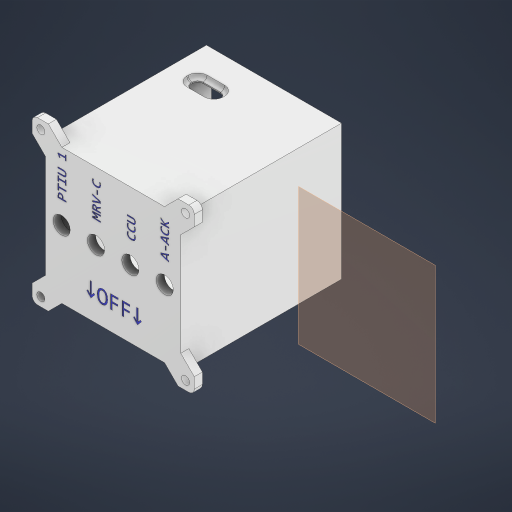
# Autodesk Inventor part: casing_1x1_lvl3
Saved by Autodesk Inventor 2024 (Build 280153000, 153)
## iProperties
Created: 2026-04-07
Part Number: casing_1x1_lvl3
Material: ABS Plastic
Document SubType Name: Modeling
Designer: schar
Density: 1.06 g/cm^3
Appearance: Smooth - White
Author: schar
Autodesk Inventor part; units mm, degrees
ref_plane "YZ Plane" through (0, 0, 0) normal (1, 0, 0) x (0, 1, 0)
sketch "Sketch1" plane through (0, 0, 0) normal (0, 0, 1) x (1, 0, 0)
  line L0 (51.6317, -54.9773) -> (91.6317, -54.9773) projected
  line L1 (85.3617, -57.4773) -> (85.3617, -57.6773) projected
  line L2 (48.6317, -97.9773) -> (48.6317, -57.9773) projected
  line L3 (91.6317, -100.9773) -> (51.6317, -100.9773) projected
  line L4 (48.6317, -77.9773) -> (85.3617, -57.5773)
  line L5 (71.6317, -54.9773) -> (71.6317, -100.9773)
  line L6 (48.5522, -54.8773) -> (94.7112, -54.8773)
  line L7 (94.7112, -54.8773) -> (94.7112, -101.0773)
  line L8 (94.7112, -101.0773) -> (48.5522, -101.0773)
  line L9 (48.5522, -101.0773) -> (48.5522, -54.8773)
  line L10 (48.5522, -54.8773) -> (94.7112, -101.0773) construction
  line L11 (94.7112, -54.8773) -> (48.5522, -101.0773) construction
  line L12 (46.6317, -52.9773) -> (96.6317, -52.9773)
  line L13 (96.6317, -52.9773) -> (96.6317, -102.9773)
  line L14 (96.6317, -102.9773) -> (46.6317, -102.9773)
  line L15 (46.6317, -102.9773) -> (46.6317, -52.9773)
  line L16 (46.6317, -52.9773) -> (96.6317, -102.9773) construction
  line L17 (96.6317, -52.9773) -> (46.6317, -102.9773) construction
  line L18 (36.6317, -42.9773) -> (106.6317, -42.9773)
  line L19 (106.6317, -42.9773) -> (106.6317, -112.9773)
  line L20 (106.6317, -112.9773) -> (36.6317, -112.9773)
  line L21 (36.6317, -112.9773) -> (36.6317, -42.9773)
  line L22 (36.6317, -42.9773) -> (106.6317, -112.9773) construction
  line L23 (106.6317, -42.9773) -> (36.6317, -112.9773) construction
  point P0 (0, 0)
  point P1 (71.6317, -77.9773)
  dimension "d0" = 46.159
  dimension "d1" = 46.2
  dimension "d2" = 50
  dimension "d3" = 50
  dimension "d4" = 70
  dimension "d5" = 70
  constraints: 40 end point, 11 midpoint, 6 parallel, 3 horizontal, 3 perpendicular
  measures "d0" distance of L7.end L8.end
  measures "d1" distance of L6.end L7.end
  measures "d2" distance of L13.end L14.end
  measures "d3" distance of L12.end L13.end
  measures "d4" distance of L19.end L20.end
  measures "d5" distance of L18.end L19.end
extrude "Extrusion1" add sketch "Sketch1" along normal blind 40 and the other way blind 30 contours L12 L13 L14 L15
ref_plane "Work Plane1" through (0, 0, 0) normal (0, 0, 1) x (1, 0, 0)
sketch "Sketch2" plane through (0, 0, 0) normal (0, 0, 1) x (1, 0, 0)
  line L0 (85.3617, -57.4773) -> (85.3617, -57.6773) projected
  circle A0 centre (51.6317, -57.9773) radius 1.1
  circle A1 centre (91.6317, -57.9773) radius 1.1
  circle A2 centre (91.6317, -97.9773) radius 1.1
  circle A3 centre (51.6317, -97.9773) radius 1.1
  line L1 (48.5522, -101.0773) -> (94.7112, -101.0773) projected
  line L2 (48.5522, -101.0773) -> (53.5522, -101.0773)
  line L3 (53.5522, -101.0773) -> (53.5522, -96.0773)
  line L4 (53.5522, -96.0773) -> (48.5522, -96.0773)
  line L5 (48.5522, -96.0773) -> (48.5522, -101.0773)
  line L6 (94.7112, -101.0773) -> (89.7112, -101.0773)
  line L7 (89.7112, -101.0773) -> (89.7112, -96.0773)
  line L8 (89.7112, -96.0773) -> (94.7112, -96.0773)
  line L9 (94.7112, -96.0773) -> (94.7112, -101.0773)
  line L10 (94.7112, -54.8773) -> (89.7112, -54.8773)
  line L11 (89.7112, -54.8773) -> (89.7112, -59.8773)
  line L12 (89.7112, -59.8773) -> (94.7112, -59.8773)
  line L13 (94.7112, -59.8773) -> (94.7112, -54.8773)
  line L14 (48.5522, -54.8773) -> (53.5522, -54.8773)
  line L15 (53.5522, -54.8773) -> (53.5522, -59.8773)
  line L16 (53.5522, -59.8773) -> (48.5522, -59.8773)
  line L17 (48.5522, -59.8773) -> (48.5522, -54.8773)
  line L18 (85.3617, -57.4773) -> (84.9017, -57.4773) projected
  line L19 (85.3617, -57.6773) -> (84.9017, -57.6773) projected
  line L20 (84.9017, -57.4773) -> (84.9017, -57.6773) projected
  point P0 (0, 0)
  point P1 (99.5, 70)
  point P2 (102.5, 113)
  point P3 (145.4592, 110.4932)
  dimension "d10" = 5
  dimension "d11" = 5
  dimension "d12" = 5
  dimension "d13" = 5
  dimension "d14" = 5
  dimension "d15" = 5
  dimension "d16" = 5
  dimension "d17" = 5
  constraints: 32 end point, 8 parallel, 4 centre point, 4 horizontal, 4 perpendicular, 1 point on line
  measures "d10" distance of L4.end L3.end
  measures "d11" distance of L3.end L2.end
  measures "d12" distance of L7.end L8.end
  measures "d13" distance of L6.end L7.end
  measures "d14" distance of L12.end L11.end
  measures "d15" distance of L11.end L10.end
  measures "d16" distance of L15.end L16.end
  measures "d17" distance of L14.end L15.end
extrude "Extrusion2" add sketch "Sketch2" along normal blind 10 contours A0 | A1 | A2 | A3 | L5 L4 L3 L1 | L7 L8 L9 L1 | L13 L12 L11 L10 | L14 L15 L16 L17
sketch "Sketch5" plane through (0, 0, 40) normal (0, 0, 1) x (1, 0, 0)
  line L0 (96.6317, -52.9773) -> (46.6317, -52.9773) projected
  line L1 (71.6317, -52.9773) -> (71.6317, -102.9773)
  line L2 (46.6317, -102.9773) -> (96.6317, -102.9773) projected
  line L3 (96.6317, -102.9773) -> (96.6317, -52.9773) projected
  line L4 (96.6317, -77.9773) -> (46.6317, -77.9773)
  line L5 (46.6317, -102.9773) -> (46.6317, -52.9773) projected
  line L6 (41.6317, -47.9773) -> (101.6317, -47.9773)
  line L7 (101.6317, -47.9773) -> (101.6317, -107.9773)
  line L8 (101.6317, -107.9773) -> (41.6317, -107.9773)
  line L9 (41.6317, -107.9773) -> (41.6317, -47.9773)
  line L10 (41.6317, -47.9773) -> (101.6317, -107.9773) construction
  line L11 (101.6317, -47.9773) -> (41.6317, -107.9773) construction
  line L12 (96.6317, -52.9773) -> (96.6317, -58.9773)
  line L13 (96.6317, -52.9773) -> (90.6317, -52.9773)
  line L14 (90.6317, -52.9773) -> (95.6317, -47.9773)
  line L15 (95.6317, -47.9773) -> (101.6317, -47.9773)
  line L16 (101.6317, -47.9773) -> (101.6317, -53.9773)
  line L17 (101.6317, -53.9773) -> (96.6317, -58.9773)
  line L18 (96.6317, -52.9773) -> (98.3995, -51.2096)
  circle A0 centre (98.3995, -51.2096) radius 1.5
  circle A1 centre (44.8639, -51.2096) radius 1.5
  line L19 (47.6317, -47.9773) -> (52.6317, -52.9773)
  line L20 (46.6317, -52.9773) -> (52.6317, -52.9773)
  line L21 (46.6317, -52.9773) -> (46.6317, -58.9773)
  line L22 (46.6317, -58.9773) -> (41.6317, -53.9773)
  line L23 (41.6317, -47.9773) -> (101.6317, -107.9773) construction
  line L24 (46.6317, -52.9773) -> (44.8639, -51.2096)
  circle A2 centre (44.8639, -104.7451) radius 1.5
  line L25 (41.6317, -101.9773) -> (46.6317, -96.9773)
  line L26 (46.6317, -102.9773) -> (46.6317, -96.9773)
  line L27 (46.6317, -102.9773) -> (52.6317, -102.9773)
  line L28 (52.6317, -102.9773) -> (47.6317, -107.9773)
  line L29 (41.6317, -107.9773) -> (101.6317, -47.9773) construction
  line L30 (46.6317, -102.9773) -> (44.8639, -104.7451)
  circle A3 centre (98.3995, -104.7451) radius 1.5
  line L31 (95.6317, -107.9773) -> (90.6317, -102.9773)
  line L32 (96.6317, -102.9773) -> (90.6317, -102.9773)
  line L33 (96.6317, -102.9773) -> (96.6317, -96.9773)
  line L34 (96.6317, -96.9773) -> (101.6317, -101.9773)
  line L35 (101.6317, -107.9773) -> (41.6317, -47.9773) construction
  line L36 (96.6317, -102.9773) -> (98.3995, -104.7451)
  point P0 (0, 0)
  point P1 (71.6317, -77.9773)
  point P2 (71.6317, -77.9773)
  point P3 (71.6317, -77.9773)
  point P4 (71.6317, -77.9773)
  point P5 (52.6317, -52.9773)
  point P6 (47.6317, -47.9773)
  point P7 (41.6317, -53.9773)
  point P8 (46.6317, -58.9773)
  point P9 (46.6317, -96.9773)
  point P10 (41.6317, -101.9773)
  point P11 (47.6317, -107.9773)
  point P12 (52.6317, -102.9773)
  point P13 (90.6317, -102.9773)
  point P14 (95.6317, -107.9773)
  point P15 (101.6317, -101.9773)
  point P16 (96.6317, -96.9773)
  dimension "d35" = 60
  dimension "d36" = 60
  dimension "d37" = 6
  dimension "d38" = 6
  dimension "d39" = 2.5
  dimension "d40" = 45
  dimension "d41" = 3
  dimension "d44" = 360
  constraints: 66 end point, 8 point on line, 7 midpoint, 6 coincident, 4 centre point, 4 parallel, 1 horizontal, 1 perpendicular, 67 other
  measures "d35" distance of L7.end L8.end
  measures "d36" distance of L6.end L7.end
  measures "d37" distance of L0.start L12.end
  measures "d38" distance of L0.start L13.end
  measures "d39" distance of L0.start L18.end
  measures "d40" angle of L17 L12
  measures "d41" diameter of A0
extrude "Extrusion5" add sketch "Sketch5" along normal blind 3 contours L3 L4 L1 L0 | L0 L14 L6 L7 L17 L3 | L1 L4 L5 L0 | L3 L2 L1 L4 | L0 L5 L22 L9 L6 L19 | L1 L2 L5 L4 | L34 L7 L8 L31 L2 L3 | L28 L8 L9 L25 L5 L2
sketch "Sketch6" plane through (0, 0, -30) normal (0, 0, -1) x (-1, 0, 0)
  line L0 (-96.6317, -102.9773) -> (-46.6317, -102.9773) projected
  line L1 (-46.6317, -102.9773) -> (-46.6317, -52.9773) projected
  line L2 (-46.6317, -52.9773) -> (-96.6317, -52.9773) projected
  line L3 (-96.6317, -52.9773) -> (-96.6317, -102.9773) projected
  line L4 (-94.7112, -54.8773) -> (-48.5522, -54.8773) projected
  line L5 (-48.5522, -54.8773) -> (-48.5522, -101.0773) projected
  line L6 (-48.5522, -101.0773) -> (-94.7112, -101.0773) projected
  line L7 (-94.7112, -101.0773) -> (-94.7112, -54.8773) projected
  line L8 (-96.6317, -52.9773) -> (-46.6317, -52.9773)
  line L9 (-46.6317, -52.9773) -> (-46.6317, -102.9773)
  line L10 (-46.6317, -102.9773) -> (-96.6317, -102.9773)
  line L11 (-96.6317, -102.9773) -> (-96.6317, -52.9773)
  point P0 (0, 0)
  constraints: 8 end point, 2 parallel, 1 horizontal, 1 perpendicular
ref_plane "Work Plane2" through (100.7, -97.28, -17.595) normal (0, 0, -1) x (0, 1, 0)
ref_plane "Work Plane3" through (99.4205, -113.1, -16.51) normal (0, 0, -1) x (0, 1, 0)
extrude "Extrusion6" cut sketch "Sketch6" against normal up to surface (13.49 mm away) contours L3 L2 L1 L0 | L4 L5 L6 L7
sketch "Sketch7" plane through (0, 0, 43) normal (0, 0, 1) x (1, 0, 0)
  line L0 (48.5522, -101.0773) -> (48.5522, -54.8773) projected
  line L1 (48.5522, -77.9773) -> (94.7112, -77.9773)
  line L2 (94.7112, -54.8773) -> (94.7112, -101.0773) projected
  line L3 (71.6317, -77.9773) -> (134.04, -77.9773)
  line L4 (48.5522, -77.9773) -> (52.5522, -77.9773)
  line L5 (94.7112, -77.9773) -> (90.7112, -77.9773)
  circle A0 centre (52.5522, -77.9773) radius 3.175
  circle A1 centre (90.7112, -77.9773) radius 3.175
  line L6 (55.7272, -77.9773) -> (117.1985, -77.9773)
  line L7 (117.1985, -77.9773) -> (127.8015, -77.9773)
  line L8 (52.5522, -77.9773) -> (65.2719, -77.9773)
  line L9 (65.2719, -77.9773) -> (77.9914, -77.9773)
  circle A2 centre (65.2719, -77.9773) radius 3.175
  circle A3 centre (77.9914, -77.9773) radius 3.175
  point P0 (0, 0)
  dimension "d56" = 6.35
  dimension "d54" = 4
  dimension "d55" = 4
  dimension "d57" = 6.35
  dimension "d60" = 12.7197
  dimension "d61" = 12.7195
  dimension "d62" = 6.35
  dimension "d63" = 6.35
  constraints: 16 end point, 8 point on line, 4 coincident, 3 centre point, 3 midpoint, 1 horizontal alignment, 2 other
  measures "d54" distance of L1.start L4.end
  measures "d55" distance of L1.end L5.end
  measures "d57" diameter of A1
  measures "d60" distance of L8.start L8.end
  measures "d61" distance of L8.end L9.end
  measures "d62" diameter of A2
  measures "d63" diameter of A3
extrude "Extrusion7" cut sketch "Sketch7" against normal blind 10
fillet "Fillet1" radius 2 4 edges at (41.6317, -47.9773, 41.5) (101.6317, -47.9773, 41.5) (101.6317, -107.9773, 41.5) (41.6317, -107.9773, 41.5)
sketch "Sketch8" plane through (52.6317, -52.9773, 43) normal (0, 1, 0) x (1, 0, 0)
  line L0 (10.19, 47.82) -> (3.81, 47.82) projected
  arc A0 (11.47, 46.54) -> (10.19, 47.82) centre (10.19, 46.54) ccw projected
  arc A1 (10.19, 44.66) -> (11.47, 45.94) centre (10.19, 45.94) ccw projected
  arc A2 (3.81, 47.82) -> (2.53, 46.54) centre (3.81, 46.54) ccw projected
  arc A3 (3.81, 47.82) -> (2.53, 46.54) centre (3.81, 46.54) ccw projected
  line L1 (2.53, 46.54) -> (2.53, 45.94) projected
  arc A4 (2.53, 45.94) -> (3.81, 44.66) centre (3.81, 45.94) ccw projected
  line L2 (3.81, 44.66) -> (6.495, 44.66) projected
  line L3 (6.495, 44.66) -> (6.495, 44.86) projected
  line L4 (6.495, 44.86) -> (3.81, 44.86) projected
  arc A5 (2.73, 45.94) -> (3.81, 44.86) centre (3.81, 45.94) ccw projected
  line L5 (2.73, 46.54) -> (2.73, 45.94) projected
  arc A6 (3.81, 47.62) -> (2.73, 46.54) centre (3.81, 46.54) ccw projected
  line L6 (3.81, 47.62) -> (10.19, 47.62) projected
  arc A7 (11.27, 46.54) -> (10.19, 47.62) centre (10.19, 46.54) ccw projected
  line L7 (11.27, 45.94) -> (11.27, 46.54) projected
  arc A8 (10.19, 44.86) -> (11.27, 45.94) centre (10.19, 45.94) ccw projected
  line L8 (6.505, 44.86) -> (10.19, 44.86) projected
  line L9 (6.505, 44.86) -> (6.505, 44.66) projected
  line L10 (6.505, 44.66) -> (10.19, 44.66) projected
  arc A9 (10.19, 44.66) -> (11.47, 45.94) centre (10.19, 45.94) ccw projected
  line L11 (11.47, 45.94) -> (11.47, 46.54) projected
  arc A10 (11.47, 46.54) -> (10.19, 47.82) centre (10.19, 46.54) ccw projected
  line L12 (10.19, 47.82) -> (3.81, 47.82) projected
  line L13 (3.75, 48.49) -> (10.25, 48.49)
  line L14 (12.25, 46.49) -> (12.25, 45.99)
  line L15 (10.25, 43.99) -> (3.75, 43.99)
  line L16 (1.75, 45.99) -> (1.75, 46.49)
  line L17 (1.75, 48.49) -> (12.25, 43.99) construction
  line L18 (12.25, 48.49) -> (1.75, 43.99) construction
  arc A11 (3.75, 48.49) -> (1.75, 46.49) centre (3.75, 46.49) ccw
  arc A12 (12.25, 46.49) -> (10.25, 48.49) centre (10.25, 46.49) ccw
  arc A13 (10.25, 43.99) -> (12.25, 45.99) centre (10.25, 45.99) ccw
  arc A14 (1.75, 45.99) -> (3.75, 43.99) centre (3.75, 45.99) ccw
  point P0 (-52.6317, 43)
  point P1 (7, 46.24)
  dimension "d67" = 10.5
  dimension "d68" = 4.5
  dimension "d69" = 2
  constraints: 12 end point, 8 point on circle, 8 point on line, 8 tangent, 4 centre point, 3 equal radius, 2 midpoint, 2 parallel, 1 horizontal, 1 perpendicular
  measures "d67" distance of L17.end L18.end
  measures "d68" distance of L18.start L17.end
  measures "d69" radius of A11
extrude "Extrusion8" cut sketch "Sketch8" against normal up to surface (1.9 mm away) contours A0 L11 A1 L10 L9 L8 A8 L7 A7 L6 A6 L5 A5 L4 L3 L2 A4 L1 A2 L0 | L13 A12 L14 A13 L15 A14 L16 A11
fillet "Fillet2" radius 1.5 8 edges at (54.9675, -52.9773, -1.5758) (54.3817, -52.9773, -3.24) (54.9675, -52.9773, -4.9042) (59.6317, -52.9773, -5.49) (64.2959, -52.9773, -4.9042) (64.8817, -52.9773, -3.24) (64.2959, -52.9773, -1.5758) (59.6317, -52.9773, -0.99) inverted yes
sketch "Sketch9" plane through (0, 0, 0) normal (0, 0, -1) x (-1, 0, 0)
  circle A0 centre (-91.5512, -58.0773) radius 1.1 projected
  circle A1 centre (-51.5512, -58.0773) radius 1.1 projected
  circle A2 centre (-51.5512, -98.0773) radius 1.1 projected
  circle A3 centre (-91.5512, -98.0773) radius 1.1 projected
  point P0 (0, 0)
extrude "Extrusion9" cut sketch "Sketch9" against normal blind 12
sketch "Sketch10" plane through (0, 0, 43) normal (0, 0, 1) x (1, 0, 0)
  line L0 (51.1902, -70.1873) -> (51.1902, -53.8905) construction
  line L1 (51.1902, -53.8905) -> (74.7807, -53.8905) construction
  line L2 (74.7807, -53.8905) -> (74.7807, -70.1873) construction
  line L3 (74.7807, -70.1873) -> (51.1902, -70.1873) construction
  line L4 (63.8972, -70.0733) -> (63.8972, -53.7765) construction
  line L5 (63.8972, -53.7765) -> (87.4877, -53.7765) construction
  line L6 (87.4877, -53.7765) -> (87.4877, -70.0733) construction
  line L7 (87.4877, -70.0733) -> (63.8972, -70.0733) construction
  line L8 (76.7751, -70.0164) -> (76.7751, -53.7195) construction
  line L9 (76.7751, -53.7195) -> (100.3657, -53.7195) construction
  line L10 (100.3657, -53.7195) -> (100.3657, -70.0164) construction
  line L11 (100.3657, -70.0164) -> (76.7751, -70.0164) construction
  line L12 (89.1835, -70.0533) -> (89.1835, -53.7564) construction
  line L13 (89.1835, -53.7564) -> (112.774, -53.7564) construction
  line L14 (112.774, -53.7564) -> (112.774, -70.0533) construction
  line L15 (112.774, -70.0533) -> (89.1835, -70.0533) construction
  line L16 (61.1991, -90.452) -> (93.6664, -90.452) construction
  line L17 (93.6664, -90.452) -> (93.6664, -103.7299) construction
  line L18 (93.6664, -103.7299) -> (61.1991, -103.7299) construction
  line L19 (61.1991, -103.7299) -> (61.1991, -90.452) construction
  spline S0 degree 2 poles (52.1386, -67.8151) (52.3244, -67.8151) (52.6906, -67.9545) (52.9803, -68.2496) (53.1607, -68.706) (53.1607, -69.0258) knots 0 0 0 1 2 3 4 4 4
  line L20 (53.1607, -69.0258) -> (53.1607, -69.4029)
  line L21 (53.1607, -69.4029) -> (54.2539, -69.4029)
  line L22 (54.2539, -69.4029) -> (54.2539, -69.8183)
  line L23 (54.2539, -69.8183) -> (51.2039, -69.8183)
  line L24 (51.2039, -69.8183) -> (51.2039, -68.9602)
  spline S1 degree 2 poles (51.2039, -68.9602) (51.2039, -68.7334) (51.305, -68.3179) (51.5291, -68.0009) (51.8844, -67.8151) (52.1386, -67.8151) knots 0 0 0 1 2 3 4 4 4
  spline S2 degree 2 poles (52.155, -68.2469) (51.8625, -68.2469) (51.5482, -68.6322) (51.5482, -68.9766) knots 0 0 0 1 2 2 2
  line L25 (51.5482, -68.9766) -> (51.5482, -69.4029)
  line L26 (51.5482, -69.4029) -> (52.8054, -69.4029)
  line L27 (52.8054, -69.4029) -> (52.8054, -69.0149)
  spline S3 degree 2 poles (52.8054, -69.0149) (52.8054, -68.6459) (52.4829, -68.2469) (52.155, -68.2469) knots 0 0 0 1 2 2 2
  line L28 (51.5592, -65.1286) -> (51.5592, -66.0332)
  line L29 (51.5592, -66.0332) -> (54.2539, -66.0332)
  line L30 (54.2539, -66.0332) -> (54.2539, -66.4541)
  line L31 (54.2539, -66.4541) -> (51.5592, -66.4541)
  line L32 (51.5592, -66.4541) -> (51.5592, -67.3587)
  line L33 (51.5592, -67.3587) -> (51.2039, -67.3587)
  line L34 (51.2039, -67.3587) -> (51.2039, -65.1286)
  line L35 (51.2039, -65.1286) -> (51.5592, -65.1286)
  line L36 (51.5537, -63.8249) -> (51.5537, -64.5273)
  line L37 (51.5537, -64.5273) -> (51.2039, -64.5273)
  line L38 (51.2039, -64.5273) -> (51.2039, -62.7017)
  line L39 (51.2039, -62.7017) -> (51.5537, -62.7017)
  line L40 (51.5537, -62.7017) -> (51.5537, -63.4041)
  line L41 (51.5537, -63.4041) -> (53.8986, -63.4041)
  line L42 (53.8986, -63.4041) -> (53.8986, -62.7017)
  line L43 (53.8986, -62.7017) -> (54.2539, -62.7017)
  line L44 (54.2539, -62.7017) -> (54.2539, -64.5273)
  line L45 (54.2539, -64.5273) -> (53.8986, -64.5273)
  line L46 (53.8986, -64.5273) -> (53.8986, -63.8249)
  line L47 (53.8986, -63.8249) -> (51.5537, -63.8249)
  spline S4 degree 2 poles (53.1907, -59.925) (53.4422, -59.925) (53.8521, -60.0671) (54.1391, -60.3431) (54.2949, -60.7421) (54.2949, -61.0018) knots 0 0 0 1 2 3 4 4 4
  spline S5 degree 2 poles (54.2949, -61.0018) (54.2949, -61.286) (54.1446, -61.6823) (53.8713, -61.931) (53.4914, -62.0458) (53.2536, -62.0458) knots 0 0 0 1 2 3 4 4 4
  line L48 (53.2536, -62.0458) -> (51.2039, -62.0458)
  line L49 (51.2039, -62.0458) -> (51.2039, -61.6304)
  line L50 (51.2039, -61.6304) -> (53.2208, -61.6304)
  spline S6 degree 2 poles (53.2208, -61.6304) (53.4012, -61.6304) (53.6718, -61.562) (53.8549, -61.409) (53.9478, -61.163) (53.9478, -60.9854) knots 0 0 0 1 2 3 4 4 4
  spline S7 degree 2 poles (53.9478, -60.9854) (53.9478, -60.6547) (53.5652, -60.3404) (53.2181, -60.3404) knots 0 0 0 1 2 2 2
  line L51 (53.2181, -60.3404) -> (51.2039, -60.3404)
  line L52 (51.2039, -60.3404) -> (51.2039, -59.925)
  line L53 (51.2039, -59.925) -> (53.1907, -59.925)
  line L54 (54.2539, -54.7159) -> (54.2539, -56.6317)
  line L55 (54.2539, -56.6317) -> (53.8767, -56.6317)
  line L56 (53.8767, -56.6317) -> (53.8767, -55.8474)
  line L57 (53.8767, -55.8474) -> (51.6494, -55.8474)
  line L58 (51.6494, -55.8474) -> (52.0456, -56.5771)
  line L59 (52.0456, -56.5771) -> (51.7013, -56.7274)
  line L60 (51.7013, -56.7274) -> (51.1902, -55.7572)
  line L61 (51.1902, -55.7572) -> (51.1902, -55.3964)
  line L62 (51.1902, -55.3964) -> (53.8767, -55.3964)
  line L63 (53.8767, -55.3964) -> (53.8767, -54.7159)
  line L64 (53.8767, -54.7159) -> (54.2539, -54.7159)
  line L65 (66.9855, -67.559) -> (66.9855, -67.9662)
  line L66 (66.9855, -67.9662) -> (65.0806, -68.0263)
  line L67 (65.0806, -68.0263) -> (64.3536, -68.0509)
  line L68 (64.3536, -68.0509) -> (64.7772, -68.193)
  line L69 (64.7772, -68.193) -> (65.9906, -68.644)
  line L70 (65.9906, -68.644) -> (65.9906, -68.9309)
  line L71 (65.9906, -68.9309) -> (64.8237, -69.36)
  line L72 (64.8237, -69.36) -> (64.3536, -69.4994)
  line L73 (64.3536, -69.4994) -> (65.1134, -69.5103)
  line L74 (65.1134, -69.5103) -> (66.9855, -69.565)
  line L75 (66.9855, -69.565) -> (66.9855, -69.9558)
  line L76 (66.9855, -69.9558) -> (63.9355, -69.8055)
  line L77 (63.9355, -69.8055) -> (63.9355, -69.3136)
  line L78 (63.9355, -69.3136) -> (65.0833, -68.9036)
  line L79 (65.0833, -68.9036) -> (65.4714, -68.7724)
  line L80 (65.4714, -68.7724) -> (65.0833, -68.644)
  line L81 (65.0833, -68.644) -> (63.9355, -68.2122)
  line L82 (63.9355, -68.2122) -> (63.9355, -67.7066)
  line L83 (63.9355, -67.7066) -> (66.9855, -67.559)
  line L84 (66.9855, -64.99) -> (66.9855, -65.4601)
  line L85 (66.9855, -65.4601) -> (66.0098, -65.9165)
  spline S8 degree 2 poles (66.0098, -65.9165) (65.8977, -65.9657) (65.7501, -66.075) (65.6654, -66.198) (65.6272, -66.3456) (65.6272, -66.4357) knots 0 0 0 1 2 3 4 4 4
  line L86 (65.6272, -66.4357) -> (65.6272, -66.6325)
  line L87 (65.6272, -66.6325) -> (66.9855, -66.6325)
  line L88 (66.9855, -66.6325) -> (66.9855, -67.0479)
  line L89 (66.9855, -67.0479) -> (63.9355, -67.0479)
  line L90 (63.9355, -67.0479) -> (63.9355, -66.2308)
  spline S9 degree 2 poles (63.9355, -66.2308) (63.9355, -65.9657) (64.053, -65.5831) (64.2634, -65.3371) (64.5586, -65.2223) (64.7389, -65.2223) knots 0 0 0 1 2 3 4 4 4
  spline S10 degree 2 poles (64.7389, -65.2223) (64.8811, -65.2223) (65.1352, -65.307) (65.3429, -65.471) (65.4932, -65.717) (65.5315, -65.8755) knots 0 0 0 1 2 3 4 4 4
  spline S11 degree 2 poles (65.5315, -65.8755) (65.5752, -65.747) (65.7966, -65.5667) (65.9825, -65.4737) knots 0 0 0 1 2 2 2
  line L91 (65.9825, -65.4737) -> (66.9855, -64.99)
  spline S12 degree 2 poles (64.7745, -65.6568) (64.5285, -65.6568) (64.2853, -65.9629) (64.2853, -66.2417) knots 0 0 0 1 2 2 2
  line L92 (64.2853, -66.2417) -> (64.2853, -66.6325)
  line L93 (64.2853, -66.6325) -> (65.2937, -66.6325)
  line L94 (65.2937, -66.6325) -> (65.2937, -66.2964)
  spline S13 degree 2 poles (65.2937, -66.2964) (65.2937, -66.1488) (65.2254, -65.9137) (65.0942, -65.747) (64.9002, -65.6568) (64.7745, -65.6568) knots 0 0 0 1 2 3 4 4 4
  line L95 (63.9355, -62.1942) -> (66.9855, -63.2327)
  line L96 (66.9855, -63.2327) -> (66.9855, -63.793)
  line L97 (66.9855, -63.793) -> (63.9355, -64.8042)
  line L98 (63.9355, -64.8042) -> (63.9355, -64.3368)
  line L99 (63.9355, -64.3368) -> (65.9906, -63.6782)
  line L100 (65.9906, -63.6782) -> (66.5946, -63.4896)
  line L101 (66.5946, -63.4896) -> (65.9906, -63.2983)
  line L102 (65.9906, -63.2983) -> (63.9355, -62.6396)
  line L103 (63.9355, -62.6396) -> (63.9355, -62.1942)
  line L104 (65.9059, -60.1745) -> (65.9059, -61.571)
  line L105 (65.9059, -61.571) -> (65.5233, -61.571)
  line L106 (65.5233, -61.571) -> (65.5233, -60.1745)
  line L107 (65.5233, -60.1745) -> (65.9059, -60.1745)
  spline S14 degree 2 poles (66.8707, -57.2338) (67.0237, -57.6) (67.0237, -58.0018) knots 0 0 0 1 1 1
  spline S15 degree 2 poles (67.0237, -58.0018) (67.0237, -58.6468) (66.2503, -59.3409) (65.4932, -59.3409) knots 0 0 0 1 2 2 2
  spline S16 degree 2 poles (65.4932, -59.3409) (65.127, -59.3409) (64.534, -59.1496) (64.1213, -58.7943) (63.8972, -58.2915) (63.8972, -57.9772) knots 0 0 0 1 2 3 4 4 4
  spline S17 degree 2 poles (63.8972, -57.9772) (63.8972, -57.7667) (63.971, -57.4005) (64.0448, -57.2338) knots 0 0 0 1 2 2 2
  line L108 (64.0448, -57.2338) -> (64.452, -57.2338)
  spline S18 degree 2 poles (64.452, -57.2338) (64.3618, -57.4005) (64.2661, -57.7558) (64.2661, -57.9635) knots 0 0 0 1 2 2 2
  spline S19 degree 2 poles (64.2661, -57.9635) (64.2661, -58.1794) (64.4274, -58.5265) (64.7335, -58.7697) (65.1735, -58.9009) (65.4577, -58.9009) knots 0 0 0 1 2 3 4 4 4
  spline S20 degree 2 poles (65.4577, -58.9009) (66.0508, -58.9009) (66.652, -58.4199) (66.652, -57.9553) knots 0 0 0 1 2 2 2
  spline S21 degree 2 poles (66.652, -57.9553) (66.652, -57.7585) (66.5618, -57.4005) (66.4799, -57.2338) knots 0 0 0 1 2 2 2
  line L109 (66.4799, -57.2338) -> (66.8707, -57.2338)
  line L110 (92.2718, -67.446) -> (92.2718, -67.8997)
  line L111 (92.2718, -67.8997) -> (91.6077, -68.1101)
  line L112 (91.6077, -68.1101) -> (91.6077, -69.3864)
  line L113 (91.6077, -69.3864) -> (92.2718, -69.5996)
  line L114 (92.2718, -69.5996) -> (92.2718, -70.0287)
  line L115 (92.2718, -70.0287) -> (89.2218, -69.0175)
  line L116 (89.2218, -69.0175) -> (89.2218, -68.4463)
  line L117 (89.2218, -68.4463) -> (92.2718, -67.446)
  line L118 (91.236, -68.2304) -> (89.6017, -68.7469)
  line L119 (89.6017, -68.7469) -> (91.236, -69.2689)
  line L120 (91.236, -69.2689) -> (91.236, -68.2304)
  line L121 (91.1922, -65.4127) -> (91.1922, -66.8092)
  line L122 (91.1922, -66.8092) -> (90.8096, -66.8092)
  line L123 (90.8096, -66.8092) -> (90.8096, -65.4127)
  line L124 (90.8096, -65.4127) -> (91.1922, -65.4127)
  line L125 (92.2718, -62.1878) -> (92.2718, -62.6414)
  line L126 (92.2718, -62.6414) -> (91.6077, -62.8519)
  line L127 (91.6077, -62.8519) -> (91.6077, -64.1282)
  line L128 (91.6077, -64.1282) -> (92.2718, -64.3414)
  line L129 (92.2718, -64.3414) -> (92.2718, -64.7704)
  line L130 (92.2718, -64.7704) -> (89.2218, -63.7592)
  line L131 (89.2218, -63.7592) -> (89.2218, -63.188)
  line L132 (89.2218, -63.188) -> (92.2718, -62.1878)
  line L133 (91.236, -62.9721) -> (89.6017, -63.4887)
  line L134 (89.6017, -63.4887) -> (91.236, -64.0107)
  line L135 (91.236, -64.0107) -> (91.236, -62.9721)
  spline S22 degree 2 poles (92.157, -59.8429) (92.31, -60.2091) (92.31, -60.6108) knots 0 0 0 1 1 1
  spline S23 degree 2 poles (92.31, -60.6108) (92.31, -61.2558) (91.5366, -61.95) (90.7796, -61.95) knots 0 0 0 1 2 2 2
  spline S24 degree 2 poles (90.7796, -61.95) (90.4133, -61.95) (89.8203, -61.7587) (89.4076, -61.4034) (89.1835, -60.9005) (89.1835, -60.5863) knots 0 0 0 1 2 3 4 4 4
  spline S25 degree 2 poles (89.1835, -60.5863) (89.1835, -60.3758) (89.2573, -60.0096) (89.3311, -59.8429) knots 0 0 0 1 2 2 2
  line L136 (89.3311, -59.8429) -> (89.7383, -59.8429)
  spline S26 degree 2 poles (89.7383, -59.8429) (89.6481, -60.0096) (89.5525, -60.3649) (89.5525, -60.5726) knots 0 0 0 1 2 2 2
  spline S27 degree 2 poles (89.5525, -60.5726) (89.5525, -60.7885) (89.7137, -61.1356) (90.0198, -61.3788) (90.4598, -61.51) (90.744, -61.51) knots 0 0 0 1 2 3 4 4 4
  spline S28 degree 2 poles (90.744, -61.51) (91.3371, -61.51) (91.9383, -61.029) (91.9383, -60.5644) knots 0 0 0 1 2 2 2
  spline S29 degree 2 poles (91.9383, -60.5644) (91.9383, -60.3676) (91.8482, -60.0096) (91.7662, -59.8429) knots 0 0 0 1 2 2 2
  line L137 (91.7662, -59.8429) -> (92.157, -59.8429)
  line L138 (92.2718, -57.0935) -> (92.2718, -57.6155)
  line L139 (92.2718, -57.6155) -> (90.7768, -58.7579)
  line L140 (90.7768, -58.7579) -> (92.2718, -58.7579)
  line L141 (92.2718, -58.7579) -> (92.2718, -59.1733)
  line L142 (92.2718, -59.1733) -> (89.2218, -59.1733)
  line L143 (89.2218, -59.1733) -> (89.2218, -58.7579)
  line L144 (89.2218, -58.7579) -> (90.6402, -58.7579)
  line L145 (90.6402, -58.7579) -> (89.2218, -57.6401)
  line L146 (89.2218, -57.6401) -> (89.2218, -57.1482)
  line L147 (89.2218, -57.1482) -> (90.6702, -58.3507)
  line L148 (90.6702, -58.3507) -> (92.2718, -57.0935)
  spline S30 degree 2 poles (79.7486, -67.6933) (79.9016, -68.0595) (79.9016, -68.4613) knots 0 0 0 1 1 1
  spline S31 degree 2 poles (79.9016, -68.4613) (79.9016, -69.1063) (79.1282, -69.8004) (78.3712, -69.8004) knots 0 0 0 1 2 2 2
  spline S32 degree 2 poles (78.3712, -69.8004) (78.005, -69.8004) (77.4119, -69.6091) (76.9992, -69.2539) (76.7751, -68.751) (76.7751, -68.4367) knots 0 0 0 1 2 3 4 4 4
  spline S33 degree 2 poles (76.7751, -68.4367) (76.7751, -68.2263) (76.8489, -67.86) (76.9227, -67.6933) knots 0 0 0 1 2 2 2
  line L149 (76.9227, -67.6933) -> (77.3299, -67.6933)
  spline S34 degree 2 poles (77.3299, -67.6933) (77.2397, -67.86) (77.1441, -68.2153) (77.1441, -68.423) knots 0 0 0 1 2 2 2
  spline S35 degree 2 poles (77.1441, -68.423) (77.1441, -68.6389) (77.3053, -68.986) (77.6114, -69.2293) (78.0514, -69.3604) (78.3356, -69.3604) knots 0 0 0 1 2 3 4 4 4
  spline S36 degree 2 poles (78.3356, -69.3604) (78.9287, -69.3604) (79.53, -68.8794) (79.53, -68.4148) knots 0 0 0 1 2 2 2
  spline S37 degree 2 poles (79.53, -68.4148) (79.53, -68.2181) (79.4398, -67.86) (79.3578, -67.6933) knots 0 0 0 1 2 2 2
  line L150 (79.3578, -67.6933) -> (79.7486, -67.6933)
  spline S38 degree 2 poles (79.7486, -65.0642) (79.9016, -65.4304) (79.9016, -65.8322) knots 0 0 0 1 1 1
  spline S39 degree 2 poles (79.9016, -65.8322) (79.9016, -66.4771) (79.1282, -67.1713) (78.3712, -67.1713) knots 0 0 0 1 2 2 2
  spline S40 degree 2 poles (78.3712, -67.1713) (78.005, -67.1713) (77.4119, -66.98) (76.9992, -66.6247) (76.7751, -66.1219) (76.7751, -65.8076) knots 0 0 0 1 2 3 4 4 4
  spline S41 degree 2 poles (76.7751, -65.8076) (76.7751, -65.5971) (76.8489, -65.2309) (76.9227, -65.0642) knots 0 0 0 1 2 2 2
  line L151 (76.9227, -65.0642) -> (77.3299, -65.0642)
  spline S42 degree 2 poles (77.3299, -65.0642) (77.2397, -65.2309) (77.1441, -65.5862) (77.1441, -65.7939) knots 0 0 0 1 2 2 2
  spline S43 degree 2 poles (77.1441, -65.7939) (77.1441, -66.0098) (77.3053, -66.3569) (77.6114, -66.6001) (78.0514, -66.7313) (78.3356, -66.7313) knots 0 0 0 1 2 3 4 4 4
  spline S44 degree 2 poles (78.3356, -66.7313) (78.9287, -66.7313) (79.53, -66.2503) (79.53, -65.7857) knots 0 0 0 1 2 2 2
  spline S45 degree 2 poles (79.53, -65.7857) (79.53, -65.5889) (79.4398, -65.2309) (79.3578, -65.0642) knots 0 0 0 1 2 2 2
  line L152 (79.3578, -65.0642) -> (79.7486, -65.0642)
  spline S46 degree 2 poles (78.8002, -62.3832) (79.0517, -62.3832) (79.4616, -62.5253) (79.7486, -62.8013) (79.9044, -63.2003) (79.9044, -63.4599) knots 0 0 0 1 2 3 4 4 4
  spline S47 degree 2 poles (79.9044, -63.4599) (79.9044, -63.7442) (79.7541, -64.1405) (79.4808, -64.3892) (79.1009, -64.5039) (78.8631, -64.5039) knots 0 0 0 1 2 3 4 4 4
  line L153 (78.8631, -64.5039) -> (76.8134, -64.5039)
  line L154 (76.8134, -64.5039) -> (76.8134, -64.0885)
  line L155 (76.8134, -64.0885) -> (78.8303, -64.0885)
  spline S48 degree 2 poles (78.8303, -64.0885) (79.0107, -64.0885) (79.2813, -64.0202) (79.4644, -63.8672) (79.5573, -63.6212) (79.5573, -63.4435) knots 0 0 0 1 2 3 4 4 4
  spline S49 degree 2 poles (79.5573, -63.4435) (79.5573, -63.1129) (79.1747, -62.7986) (78.8276, -62.7986) knots 0 0 0 1 2 2 2
  line L156 (78.8276, -62.7986) -> (76.8134, -62.7986)
  line L157 (76.8134, -62.7986) -> (76.8134, -62.3832)
  line L158 (76.8134, -62.3832) -> (78.8002, -62.3832)
  line L159 (64.4383, -93.7898) -> (64.8639, -94.1616)
  line L160 (64.8639, -94.1616) -> (63.3541, -95.9045)
  line L161 (63.3541, -95.9045) -> (61.8442, -94.1616)
  line L162 (61.8442, -94.1616) -> (62.2699, -93.7898)
  line L163 (62.2699, -93.7898) -> (63.0897, -94.8158)
  line L164 (63.0897, -94.8158) -> (63.0629, -94.1079)
  line L165 (63.0629, -94.1079) -> (63.0629, -90.452)
  line L166 (63.0629, -90.452) -> (63.6453, -90.452)
  line L167 (63.6453, -90.452) -> (63.6453, -94.1079)
  line L168 (63.6453, -94.1079) -> (63.6229, -94.8158)
  line L169 (63.6229, -94.8158) -> (64.4383, -93.7898)
  spline S50 degree 2 poles (69.6086, -93.3014) (69.6086, -93.9779) (69.2905, -94.9546) (68.7528, -95.5953) (68.027, -95.9045) (67.6283, -95.9045) knots 0 0 0 1 2 3 4 4 4
  spline S51 degree 2 poles (67.6283, -95.9045) (67.1444, -95.9045) (66.4276, -95.555) (65.9571, -94.8964) (65.7286, -93.9511) (65.7286, -93.3597) knots 0 0 0 1 2 3 4 4 4
  spline S52 degree 2 poles (65.7286, -93.3597) (65.7286, -92.6921) (66.0423, -91.7154) (66.5799, -91.0747) (67.3012, -90.7656) (67.7044, -90.7656) knots 0 0 0 1 2 3 4 4 4
  spline S53 degree 2 poles (67.7044, -90.7656) (68.1838, -90.7656) (68.9007, -91.1195) (69.3756, -91.7736) (69.6086, -92.7145) (69.6086, -93.3014) knots 0 0 0 1 2 3 4 4 4
  spline S54 degree 2 poles (68.9276, -93.3507) (68.9276, -92.9116) (68.7887, -92.1813) (68.484, -91.6527) (68.0046, -91.3615) (67.6641, -91.3615) knots 0 0 0 1 2 3 4 4 4
  spline S55 degree 2 poles (67.6641, -91.3615) (67.3371, -91.3615) (66.8621, -91.6706) (66.5575, -92.2037) (66.4096, -92.9206) (66.4096, -93.3238) knots 0 0 0 1 2 3 4 4 4
  spline S56 degree 2 poles (66.4096, -93.3238) (66.4096, -93.7674) (66.5485, -94.4977) (66.8532, -95.0218) (67.3281, -95.3131) (67.6641, -95.3131) knots 0 0 0 1 2 3 4 4 4
  spline S57 degree 2 poles (67.6641, -95.3131) (67.9912, -95.3131) (68.4706, -95.0039) (68.7797, -94.4708) (68.9276, -93.7584) (68.9276, -93.3507) knots 0 0 0 1 2 3 4 4 4
  line L170 (73.4213, -91.4197) -> (71.2976, -91.4197)
  line L171 (71.2976, -91.4197) -> (71.2976, -93.0416)
  line L172 (71.2976, -93.0416) -> (73.3093, -93.0416)
  line L173 (73.3093, -93.0416) -> (73.3093, -93.6106)
  line L174 (73.3093, -93.6106) -> (71.2976, -93.6106)
  line L175 (71.2976, -93.6106) -> (71.2976, -95.8373)
  line L176 (71.2976, -95.8373) -> (70.6032, -95.8373)
  line L177 (70.6032, -95.8373) -> (70.6032, -90.8373)
  line L178 (70.6032, -90.8373) -> (73.4213, -90.8373)
  line L179 (73.4213, -90.8373) -> (73.4213, -91.4197)
  line L180 (77.7313, -91.4197) -> (75.6077, -91.4197)
  line L181 (75.6077, -91.4197) -> (75.6077, -93.0416)
  line L182 (75.6077, -93.0416) -> (77.6193, -93.0416)
  line L183 (77.6193, -93.0416) -> (77.6193, -93.6106)
  line L184 (77.6193, -93.6106) -> (75.6077, -93.6106)
  line L185 (75.6077, -93.6106) -> (75.6077, -95.8373)
  line L186 (75.6077, -95.8373) -> (74.9132, -95.8373)
  line L187 (74.9132, -95.8373) -> (74.9132, -90.8373)
  line L188 (74.9132, -90.8373) -> (77.7313, -90.8373)
  line L189 (77.7313, -90.8373) -> (77.7313, -91.4197)
  line L190 (81.6785, -93.7898) -> (82.1041, -94.1616)
  line L191 (82.1041, -94.1616) -> (80.5942, -95.9045)
  line L192 (80.5942, -95.9045) -> (79.0844, -94.1616)
  line L193 (79.0844, -94.1616) -> (79.51, -93.7898)
  line L194 (79.51, -93.7898) -> (80.3299, -94.8158)
  line L195 (80.3299, -94.8158) -> (80.303, -94.1079)
  line L196 (80.303, -94.1079) -> (80.303, -90.452)
  line L197 (80.303, -90.452) -> (80.8854, -90.452)
  line L198 (80.8854, -90.452) -> (80.8854, -94.1079)
  line L199 (80.8854, -94.1079) -> (80.863, -94.8158)
  line L200 (80.863, -94.8158) -> (81.6785, -93.7898)
  point P0 (0, 0)
  constraints: 10 other
extrude "Extrusion10" cut sketch "Sketch10" against normal blind 0.2
thread "Thread1" size "M2.2x0.45" class "6H" standard "ANSI Metric M Profile" length 15.103
thread "Thread2" size "M2.2x0.45" class "6H" standard "ANSI Metric M Profile" length 15.103
thread "Thread3" size "M2.2x0.45" class "6H" standard "ANSI Metric M Profile" length 15.103
thread "Thread4" size "M2.2x0.45" class "6H" standard "ANSI Metric M Profile" length 15.103
body "Solid1"
